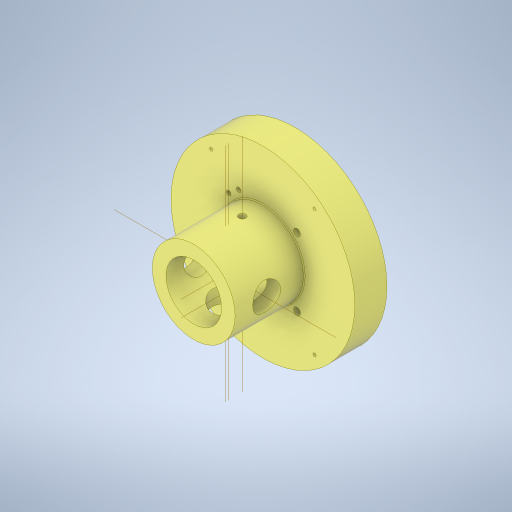
# Autodesk Inventor part: Insulation_4
Saved by Autodesk Inventor 2023 (Build 270158030, 158C)
## iProperties
Created: 2019-02-15
Part Number: Insulation_4
Material: ABS Plastic
Document SubType Name: Modeling
Designer: rainer
Density: 1.06 g/cm^3
Appearance: Smooth - White
Author: rainer
Autodesk Inventor part; units mm, degrees
ref_plane "YZ Plane" through (0, 0, 0) normal (1, 0, 0) x (0, 1, 0)
ref_plane "XZ Plane" through (0, 0, 0) normal (0, 1, 0) x (-1, 0, 0)
ref_plane "XY Plane" through (0, 0, 0) normal (0, 0, 1) x (1, 0, 0)
sketch "Sketch1" plane through (0, 0, 0) normal (0, 0, 1) x (1, 0, 0)
  circle A0 centre (0, 0) radius 119
  dimension "d0" = 238
  constraints: 1 centre point, 1 coincident
  measures "d0" diameter of A0
extrude "Extrusion1" add sketch "Sketch1" along normal blind 50
sketch "Sketch2" plane through (0, 0, 50) normal (0, 0, 1) x (1, 0, 0)
  circle A0 centre (0, 0) radius 200
  dimension "d3" = 400
  constraints: 1 centre point, 1 coincident
  measures "d3" diameter of A0
extrude "Extrusion2" add sketch "Sketch2" along normal blind 70
sketch "Sketch3" plane through (0, 0, 120) normal (0, 0, 1) x (1, 0, 0)
  circle A0 centre (0, 0) radius 90
  dimension "d6" = 180
  constraints: 1 centre point, 1 coincident
  measures "d6" diameter of A0
extrude "Extrusion3" add sketch "Sketch3" along normal blind 150
sketch "Sketch4" plane through (0, 0, 270) normal (0, 0, 1) x (1, 0, 0)
  circle A0 centre (0, 0) radius 60.5
  dimension "d9" = 121
  constraints: 1 centre point, 1 coincident
  measures "d9" diameter of A0
extrude "Extrusion4" cut sketch "Sketch4" against normal blind 180
sketch "Sketch5" plane through (0, 0, 90) normal (0, 0, 1) x (1, 0, 0)
  circle A0 centre (0, 0) radius 30.5
  dimension "d12" = 61
  constraints: 1 centre point, 1 coincident
  measures "d12" diameter of A0
extrude "Extrusion5" cut sketch "Sketch5" against normal blind 180
sketch "Sketch6" plane through (0, 0, 50) normal (0, 0, -1) x (-1, 0, 0)
  circle A0 centre (0, 0) radius 129
  circle A1 centre (0, 0) radius 139
  dimension "d15" = 258
  dimension "d16" = 278
  constraints: 2 centre point, 2 coincident
  measures "d15" diameter of A0
  measures "d16" diameter of A1
extrude "Extrusion6" add sketch "Sketch6" along normal blind 20
fillet "Fillet1" radius 2 3 edges at (139, 0, 30) (129, 0, 30) (-119, 0, 0)
chamfer "Chamfer1" distance 10 angle 10 1 edges at (-119, 0, 50) measured on face at (-119, 0, 49.5)
fillet "Fillet2" radius 2 1 edges at (139, 0, 50)
sketch "Sketch7" plane through (0, 0, 0) normal (0, 0, -1) x (-1, 0, 0)
  circle A0 centre (0, -35) radius 3.5
  line L0 (-3.5, -30) -> (3.5, -30)
  line L1 (3.5, -30) -> (3.5, -35)
  line L2 (3.5, -35) -> (-3.5, -35)
  line L3 (-3.5, -35) -> (-3.5, -30)
  point P0 (0, 0)
  point P1 (0, -30)
  dimension "d24" = 7
  dimension "d25" = 35
  dimension "d26" = 7
  dimension "d27" = 30
  dimension "d28" = 5
  constraints: 8 end point, 2 parallel, 1 centre point, 1 horizontal, 1 midpoint, 1 perpendicular, 1 vertical alignment
  measures "d24" diameter of A0
  measures "d25" distance of point (0, 0) A0.centre
  measures "d26" distance of L0.start L0.end
  measures "d27" distance from line of point (0, 0) L0
  measures "d28" distance of L2.end L0.start
extrude "Extrusion7" cut sketch "Sketch7" against normal blind 180
fillet "Fillet3" radius 2 2 edges at (-3.5, -30.2985, 45) (3.5, -30.2985, 45)
fillet "Fillet5" radius 2 1 edges at (-90, 0, 120)
sketch "Sketch8" plane through (0, 0, 0) normal (0, 0, -1) x (-1, 0, 0)
  circle A0 centre (0, 0) radius 105
  line L0 (0, 0) -> (-74.2462, 74.2462)
  line L1 (0, 0) -> (105, 0) construction
  line L2 (0, 0) -> (74.2462, 74.2462)
  line L3 (0, 0) -> (105, 0) construction
  line L4 (0, 0) -> (52.5, 90.9327)
  line L5 (0, 0) -> (105, 0) construction
  line L6 (-74.2462, 74.2462) -> (-74.2462, -74.2462)
  line L7 (0, 0) -> (80.4347, -67.4927)
  line L8 (0, 0) -> (105, 0) construction
  point P0 (-71.1426, 70.7811)
  point P1 (-57.5683, 72.0634)
  dimension "d34" = 210
  dimension "d35" = 105
  dimension "d36" = 135
  dimension "d37" = 105
  dimension "d38" = 45
  dimension "d48" = 105
  dimension "d49" = 60
  dimension "d87" = 105
  dimension "d88" = 40
  constraints: 18 end point, 4 coincident, 4 equal length, 4 horizontal, 2 point on circle, 1 centre point, 1 perpendicular, 1 point on line, 1 vertical
  measures "d34" diameter of A0
  measures "d35" distance of L0.start L0.end
  measures "d36" angle of L1 L0
  measures "d37" distance of L0.start L2.end
  measures "d38" angle of L3 L2
  measures "d48" distance of L0.start L4.end
  measures "d49" angle of L5 L4
  measures "d87" distance of L0.start L7.end
  measures "d88" angle of L7 L8
hole "Hole1" at (-74.2462, 74.2462, 0) at (-80.4347, -67.4927, 0) direction (0, 0, 1) diameter 10 end through all
thicken "Thicken1" operation add thickness 0.5 both sides no extend neighbours yes toward (0, 0, 1) faces at (-79.9254, 1.8077, 270)
sketch "Sketch9" plane through (0, 0, 0) normal (0, 0, -1) x (-1, 0, 0)
  circle A0 centre (0, 0) radius 105
  line L0 (0, 0) -> (52.5, 90.9327)
  line L1 (0, 0) -> (105, 0) construction
  dimension "d50" = 210
  dimension "d51" = 105
  dimension "d52" = 60
  constraints: 4 end point, 2 coincident, 1 centre point, 1 equal length, 1 horizontal
  measures "d50" diameter of A0
  measures "d51" distance of L0.start L0.end
  measures "d52" angle of L1 L0
hole "Hole2" at (-52.5, 90.9327, 0) direction (0, 0, 1) diameter 10 end through all
sketch "Sketch10" plane through (0, 0, 0) normal (1, 0, 0) x (0, 1, 0)
  circle A0 centre (0, 201.8) radius 30.25
  line L0 (90, 270.5) -> (-90, 270.5) projected
  point P0 (0, 0)
  dimension "d60" = 60.5
  dimension "d61" = 68.7
  constraints: 1 centre point
  measures "d60" diameter of A0
  measures "d61" distance from line of L0 A0.centre
extrude "Extrusion8" cut sketch "Sketch10" along normal mid plane 400
sketch "Sketch11" plane through (0, 0, 0) normal (0, 1, 0) x (-1, 0, 0)
  circle A0 centre (0, 165) radius 7.5
  line L0 (90, 270.5) -> (-90, 270.5) projected
  point P0 (0, 0)
  dimension "d64" = 15
  dimension "d65" = 105.5
  constraints: 1 centre point
  measures "d64" diameter of A0
  measures "d65" distance from line of L0 A0.centre
extrude "Extrusion9" cut sketch "Sketch11" along normal blind 400
sketch "Sketch12" plane through (0, 0, 0) normal (0, 1, 0) x (-1, 0, 0)
  circle A0 centre (0, 195) radius 35
  line L0 (90, 270.5) -> (-90, 270.5) projected
  point P0 (0, 0)
  dimension "d68" = 70
  dimension "d69" = 75.5
  constraints: 1 centre point
  measures "d68" diameter of A0
  measures "d69" distance from line of L0 A0.centre
extrude "Extrusion10" cut sketch "Sketch12" against normal blind 400
sketch "Sketch14" plane through (0, 0, 120) normal (0, 0, 1) x (1, 0, 0)
  circle A0 centre (0, 0) radius 155 projected
  circle A1 centre (137.5001, 112.4999) radius 2.4585
  circle A2 centre (137.4999, -112.5001) radius 2.4585 projected
  circle A3 centre (-137.5001, -112.4999) radius 2.4585 projected
  circle A4 centre (-137.4999, 112.5001) radius 2.4585 projected
  circle A5 centre (112.5001, 137.4999) radius 2.4585 projected
  circle A6 centre (112.4999, -137.5001) radius 2.4585 projected
  circle A7 centre (-112.5001, -137.4999) radius 2.4585 projected
  circle A8 centre (-112.4999, 137.5001) radius 2.4585 projected
  point P0 (0, 0)
  point P1 (137.0879, -110.9866)
  point P2 (-138.9557, -112.5538)
  constraints: 1 centre point
hole "Hole3" at (-112.4999, 137.5001, 120) at (112.5001, 137.4999, 120) at (112.4999, -137.5001, 120) at (-112.5001, -137.4999, 120) direction (0, 0, -1) diameter 6.6 end through all clearance for "Socket Head Cap Screw ISO 4762" size "M6" standard "ISO"
hole "Hole4" at (74.2462, 74.2462, 0) at (74.2462, -74.2462, 0) direction (0, 0, 1) diameter 15 end through all
ref_plane "Work Plane1" through (0, 0, 201.8) normal (0, 0, 1) x (1, 0, 0)
body "Solid1"
